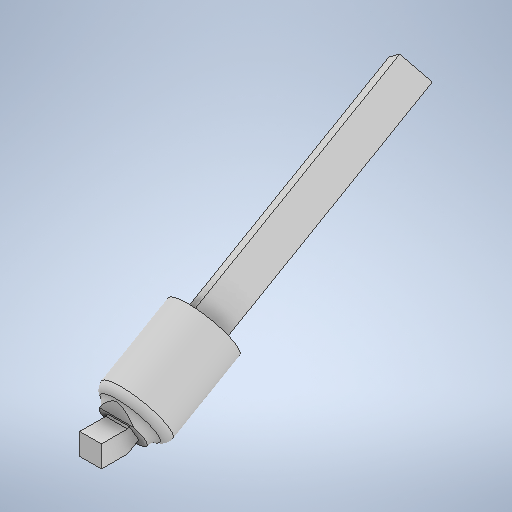
# Autodesk Inventor part: Bras hélice
Saved by Autodesk Inventor 2026.2 (Build 302298010, 298A)
## iProperties
Created: 2026-04-02
Part Number: Bras hélice
Material: Générique
Document SubType Name: Modeling
Designer: Genon
Density: 1 g/cm^3
Appearance: Par défaut
Author: Genon
Autodesk Inventor part; units mm, degrees
ref_plane "YZ Plane" through (0, 0, 0) normal (1, 0, 0) x (0, 1, 0)
sketch "Esquisse1" plane through (0, 0, 0) normal (0, 0, 1) x (1, 0, 0)
  line L0 (0, 0) -> (5, 0)
  line L1 (5, 0) -> (5, 5)
  line L2 (5, 5) -> (0, 5)
  line L3 (0, 5) -> (0, 0)
  dimension "d0" = 5
  dimension "d1" = 5
  constraints: 8 end point, 2 parallel, 1 horizontal, 1 perpendicular
  measures "d0" distance of L2.end L1.end
  measures "d1" distance of L1.end L0.end
extrude "Extrusion1" add sketch "Esquisse1" along normal blind 5
ref_plane "Plan de construction1" through (0, 0, 5) normal (0, -0.5, 0.8660254) x (1, 0, 0)
sketch "Esquisse2" plane through (0, 0, 5) normal (0, -0.5, 0.8660254) x (1, 0, 0)
  line L0 (0, 4.3301) -> (5, 4.3301)
  line L1 (5, 0) -> (5, 4.3301) projected
  line L2 (0, 4.3301) -> (5, 4.3301)
  line L3 (5, 4.3301) -> (5, 0)
  line L4 (5, 0) -> (0, 0)
  line L5 (0, 0) -> (0, 4.3301)
  point P0 (0, -2.5)
  constraints: 10 end point, 2 horizontal, 2 parallel, 1 perpendicular
extrude "Extrusion2" add sketch "Esquisse2" along normal mid plane 5
sketch "Esquisse3" plane through (0, -1.25, 7.1651) normal (0, -0.5, 0.8660254) x (1, 0, 0)
  line L0 (0, 0) -> (5, 0) projected
  line L1 (5, 0) -> (5, 4.3301) projected
  line L2 (5, 4.3301) -> (0, 4.3301) projected
  line L3 (0, 4.3301) -> (0, 0) projected
  point P0 (0, -2.5)
extrude "Extrusion3" add sketch "Esquisse3" along normal blind 5
fillet "Congé1" radius 2 2 edges at (2.5, 0, 13.6603) (2.5, -3.75, 11.4952)
ref_plane "Plan de construction2" through (5, 5, 0) normal (0, 0.5, -0.8660254) x (-1, 0, 0)
sketch "Esquisse4" plane through (5, 5, 0) normal (0, 0.5, -0.8660254) x (-1, 0, 0)
  line L0 (0, 0) -> (0, 2.5) projected
  line L1 (5, -4.3301) -> (5, -1.8301) projected
  line L2 (0, 0) -> (5, 0)
  line L3 (5, 0) -> (5, -4.3301)
  line L4 (5, -4.3301) -> (0, -4.3301)
  line L5 (0, -4.3301) -> (0, 0)
  point P0 (5, -1.8301)
  constraints: 8 end point, 2 parallel, 1 horizontal, 1 perpendicular
extrude "Extrusion4" add sketch "Esquisse4" along normal mid plane 5
sketch "Esquisse6" plane through (5, 6.25, -2.1651) normal (0, 0.5, -0.8660254) x (-1, 0, 0)
  line L0 (0, 0) -> (5, 0) projected
  line L1 (5, 0) -> (2.5, 0)
  line L2 (2.5, 0) -> (2.5, -2.165)
  circle A0 centre (2.5, -2.165) radius 5
  point P0 (5, -4.3301)
  dimension "d14" = 2.165
  dimension "d15" = 10
  constraints: 4 end point, 1 centre point, 1 coincident, 1 midpoint, 1 vertical
  measures "d14" distance of L1.end L2.end
  measures "d15" diameter of A0
extrude "Extrusion5" add sketch "Esquisse6" against normal blind 2
sketch "Esquisse7" plane through (5, 5, 5) normal (1, 0, 0) x (0, 0, -1)
  line L0 (5.433, 0.25) -> (5, 0) projected
  line L1 (5, 0) -> (-0.081, 0)
  line L2 (-0.081, 0) -> (-0.081, 15.1439)
  line L3 (-0.081, 15.1439) -> (5, 15.1439)
  line L4 (5, 15.1439) -> (5, 0)
  point P0 (5, -5)
  constraints: 8 end point, 2 parallel, 1 horizontal, 1 perpendicular
extrude "Extrusion6" cut sketch "Esquisse7" along normal through all both and the other way through all
sketch "Esquisse8" plane through (2.5, 4.3751, -3.2476) normal (0, 0.5, -0.8660254) x (-1, 0, 0)
  arc A0 (3.9765, 3.031) -> (-3.9765, 3.031) centre (0, 0) ccw projected
  line L0 (0, 5) -> (-5, 0)
  arc A1 (-3.9765, 3.031) -> (3.9765, 3.031) centre (0, 0) ccw projected
  line L1 (0, -5) -> (-5, 0)
  line L2 (0, -5) -> (5, 0)
  line L3 (5, 0) -> (0, 5)
  point P0 (2.5, -2.1651)
  constraints: 8 end point, 4 point on circle, 3 perpendicular
extrude "Extrusion7" add sketch "Esquisse8" along normal blind 74.5 contours L3 L2 L1 L0
sketch "Esquisse9" plane through (5, 6.25, -2.1651) normal (0, 0.5, -0.8660254) x (-1, 0, 0)
  line L0 (7.5, -2.165) -> (2.5, 2.835) projected
  arc A0 (-1.4765, 0.866) -> (6.4765, 0.866) centre (2.5, -2.165) ccw projected
  arc A1 (6.4765, 0.866) -> (-1.4765, 0.866) centre (2.5, -2.165) ccw projected
  circle A2 centre (2.5, -2.165) radius 7.5
  point P0 (5, -4.3301)
  dimension "d24" = 15
  constraints: 1 centre point, 1 coincident
  measures "d24" diameter of A2
extrude "Extrusion8" add sketch "Esquisse9" along normal blind 19.5 contours A0 A1 L0 | L0 A1 A0 | A2
fillet "Congé2" radius 2 1 edges at (7.5, 4.3751, -3.2476)
fillet "Congé3" radius 2 1 edges at (10, 4.3751, -3.2476)
sketch "Esquisse10" plane through (5, 5, 5) normal (1, 0, 0) x (0, 0, -1)
  line L0 (0, 0) -> (-6.9282, -4) projected
  line L1 (0, 0) -> (-8.5321, 0)
  line L2 (-8.5321, 0) -> (-8.5321, -9.6747)
  line L3 (-8.5321, -9.6747) -> (0, -9.6747)
  line L4 (0, -9.6747) -> (0, 0)
  point P0 (5, -5)
  constraints: 8 end point, 2 parallel, 1 horizontal, 1 perpendicular
extrude "Extrusion9" cut sketch "Esquisse10" against normal through all
sketch "Esquisse11" plane through (5, 0, 5) normal (0, 0, 1) x (1, 0, 0)
  line L0 (-5, 0) -> (0, 0) projected
  line L1 (0, 5) -> (0, 0) projected
  line L2 (0, 5) -> (-5, 5) projected
  line L3 (-5, 0) -> (-5, 5) projected
  line L4 (-5, 0) -> (0, 0) projected
  line L5 (0, 5) -> (0, 0) projected
  line L6 (0, 5) -> (-5, 5) projected
  line L7 (-5, 0) -> (-5, 5) projected
extrude "Extrusion10" add sketch "Esquisse11" along normal blind 1
